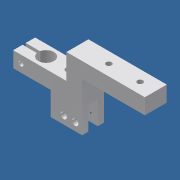
# Autodesk Inventor part: J001396
Saved by Autodesk Inventor 2012 SP2 (Build 160219200, 219)
## iProperties
Created: 2012-04-07
Part Number: J001396
Material: ALUMINUM, 6061-T651
Document SubType Name: Modeling
Designer: Igor
Density: 2.7 g/cm^3
Mass: 74.0538 g
Surface Area: 93.0623 cm^2
Volume: 27.4273 cm^3
Project: P-51601
Description: HEATER HOLDER
Vendor: HHMI: JFRC - ID&F
SPECIAL FINISH: ANODIZE PER MIL-A-8625F, TYPE II, CLASS 2 (BLACK)
ALTERED ITEM PART NUMBER: N/A
ALTERED ITEM VENDOR: N/A
DESIGN DEPARTMENT: HHMI: JFRC - ID&F
LAB/DEPT: GONEN (LAB)
REQUESTING SCIENTIST: GONEN, TAMIR
SURFACE ROUGHNESS: 32 Ra
ALTERED ITEM DESCRIPTION: N/A
Author: Igor
Revision Number: -
Autodesk Inventor part; units mm, degrees
note: some values were not read from the file. Chosen so that the rebuilt part matches the saved one: direction of "Hole3"; direction of "Hole6".
ref_plane "YZ Plane" through (0, 0, 0) normal (1, 0, 0) x (0, 1, 0)
ref_plane "XZ Plane" through (0, 0, 0) normal (0, 1, 0) x (-1, 0, 0)
ref_plane "XY Plane" through (0, 0, 0) normal (0, 0, 1) x (1, 0, 0)
sketch "Sketch1" plane through (0, 0, 0) normal (0, 0, 1) x (1, 0, 0)
  line L0 (0, 0) -> (63.5, 0)
  line L1 (63.5, 0) -> (63.5, -12.7)
  line L2 (63.5, -12.7) -> (12.7, -12.7)
  line L3 (12.7, -12.7) -> (12.7, -33.02)
  line L4 (12.7, -33.02) -> (-43.18, -33.02)
  line L5 (-43.18, -33.02) -> (-43.18, -20.32)
  line L6 (-43.18, -20.32) -> (0, -20.32)
  line L7 (0, -20.32) -> (0, 0)
  dimension "d0" = 12.7
  dimension "d2" = 12.7
  dimension "d3" = 12.7
  dimension "d4" = 43.18
  dimension "d5" = 20.32
  dimension "d22" = 50.8
  constraints: 16 end point, 6 parallel, 1 horizontal, 1 perpendicular
  measures "d0" distance of L0.end L1.end
  measures "d2" distance between parallel lines of L3 L7
  measures "d3" distance of L4.end L5.end
  measures "d4" distance between parallel lines of L7 L5
  measures "d5" distance of L6.end L0.start
  measures "d22" distance between parallel lines of L1 L3
extrude "Extrusion1" add sketch "Sketch1" along normal blind 17.78
sketch "Sketch2" plane through (0, 0, 0) normal (0, 1, 0) x (1, 0, 0)
  line L0 (63.5, 0) -> (63.5, -17.78) projected
  line L1 (0, 0) -> (0, -17.78) projected
  line L2 (0, -8.89) -> (63.5, -8.89) construction
  point P0 (50.8, -8.89)
  point P1 (25.4, -8.89)
  dimension "d8" = 12.7
  dimension "d9" = 25.4
  constraints: 2 end point, 2 midpoint, 2 point on line
  measures "d8" distance from line of L0 point (50.8, -8.89)
  measures "d9" distance of point (25.4, -8.89) point (50.8, -8.89)
hole "Hole1" at (50.8, 0, 8.89) at (25.4, 0, 8.89) direction (0, -1, 0) diameter 4.4958 end through all clearance for "Flat Head Machine Screw (82)" size "#8" standard "Ansi Unified Screw Threads"
sketch "Sketch3" plane through (-43.18, -33.02, 0) normal (0, -1, 0) x (1, 0, 0)
  line L0 (0, 0) -> (0, 17.78) projected
  line L1 (55.88, 0) -> (55.88, 17.78) projected
  line L2 (0, 8.89) -> (55.88, 8.89) construction
  arc A0 (11.5583, 7.62) -> (11.5583, 10.16) centre (17.78, 8.89) ccw
  line L3 (11.5583, 10.16) -> (0, 10.16)
  line L4 (0, 7.62) -> (11.5583, 7.62)
  line L5 (0, 10.16) -> (0, 7.62)
  point P0 (43.18, 0)
  dimension "d17" = 12.7
  dimension "d18" = 17.78
  dimension "d19" = 2.54
  constraints: 8 end point, 3 point on line, 2 midpoint, 2 point on circle, 1 centre point, 1 collinear, 1 parallel, 1 perpendicular, 1 other
  measures "d17" diameter of A0
  measures "d18" distance from line of L0 A0.centre
  measures "d19" distance between parallel lines of L4 L3
extrude "Extrusion2" cut sketch "Sketch3" against normal up to next
sketch "Sketch4" plane through (0, 0, 17.78) normal (0, 0, 1) x (1, 0, 0)
  line L0 (-43.18, -33.02) -> (-43.18, -20.32) projected
  line L1 (12.7, -12.7) -> (12.7, -33.02) projected
  line L2 (-43.18, -26.67) -> (12.7, -26.67) construction
  point P0 (-36.83, -26.67)
  dimension "d23" = 6.35
  constraints: 2 end point, 2 point on line, 1 midpoint, 1 perpendicular
  measures "d23" distance from line of point (-36.83, -26.67) L0
hole "Hole3" at (-36.83, -26.67, 17.78) direction (0, 0, -1) diameter 3.81 end up to surface clearance for "Flat Head Machine Screw (82)" size "#6" standard "Ansi Unified Screw Threads"
hole "Hole4" at (-36.83, -26.67, 17.78) direction (0, 0, -1) diameter 2.6416 end through all thread size "6-32 UNC" class "2B" standard "ANSI Unified Screw Threads"
sketch "Sketch6" plane through (-43.18, -33.02, 0) normal (0, -1, 0) x (1, 0, 0)
  line L0 (0, 10.16) -> (11.5583, 10.16) projected
  arc A0 (11.5583, 7.62) -> (11.5583, 10.16) centre (17.78, 8.89) ccw projected
  line L1 (11.5583, 7.62) -> (0, 7.62) projected
  line L2 (0, 0) -> (0, 7.62) projected
  line L3 (55.88, 0) -> (0, 0) projected
  line L4 (55.88, 0) -> (55.88, 17.78) projected
  line L5 (55.88, 17.78) -> (0, 17.78) projected
  line L6 (0, 10.16) -> (0, 17.78) projected
  line L7 (55.88, 17.78) -> (30.48, 17.78)
  line L8 (30.48, 17.78) -> (30.48, 12.7)
  line L9 (30.48, 12.7) -> (55.88, 12.7)
  line L10 (55.88, 12.7) -> (55.88, 17.78)
  line L11 (55.88, 0) -> (30.48, 0)
  line L12 (30.48, 0) -> (30.48, 5.08)
  line L13 (30.48, 5.08) -> (55.88, 5.08)
  line L14 (55.88, 5.08) -> (55.88, 0)
  point P0 (43.18, 0)
  dimension "d56" = 5.08
  dimension "d57" = 25.4
  dimension "d58" = 5.08
  dimension "d59" = 25.4
  constraints: 16 end point, 4 parallel, 2 horizontal, 2 perpendicular
  measures "d56" distance of L9.end L4.end
  measures "d57" distance between parallel lines of L8 L4
  measures "d58" distance between parallel lines of L3 L13
  measures "d59" distance between parallel lines of L12 L14
extrude "Extrusion3" add sketch "Sketch6" along normal blind 19.05 contours L5 L4 L9 L8 | L12 L13 L4 L3
sketch "Sketch8" plane through (0, 0, 17.78) normal (0, 0, 1) x (1, 0, 0)
  line L0 (-12.7, -33.02) -> (-43.18, -33.02) projected
  line L1 (12.7, -12.7) -> (12.7, -52.07) projected
  point P0 (0, 0)
  point P1 (7.112, -45.72)
  point P2 (-2.286, -45.72)
  dimension "d66" = 12.7
  dimension "d67" = 12.7
  dimension "d68" = 14.986
  dimension "d69" = 9.398
  measures "d66" distance from line of L0 point (-2.286, -45.72)
  measures "d67" distance from line of L0 point (7.112, -45.72)
  measures "d68" distance from line of point (-2.286, -45.72) L1
  measures "d69" distance of point (7.112, -45.72) point (-2.286, -45.72)
hole "Hole6" at (7.112, -45.72, 17.78) at (-2.286, -45.72, 17.78) direction (0, 0, -1) diameter 5.08 end up to surface
hole "Hole7" at (-2.286, -45.72, 17.78) direction (0, 0, -1) diameter 1.7018 end through all
hole "Hole8" at (7.112, -45.72, 17.78) direction (0, 0, -1) diameter 1.7018 end through all
sketch "Sketch9" plane through (-43.18, -20.32, 0) normal (0, 1, 0) x (1, 0, 0)
  line L0 (11.5583, -10.16) -> (0, -10.16) projected
  line L1 (0, -10.16) -> (0, -17.78) projected
  line L2 (0, -17.78) -> (43.18, -17.78) projected
  line L3 (43.18, 0) -> (43.18, -17.78) projected
  line L4 (0, 0) -> (43.18, 0) projected
  line L5 (0, 0) -> (0, -7.62) projected
  line L6 (0, -7.62) -> (11.5583, -7.62) projected
  arc A0 (11.5583, -10.16) -> (11.5583, -7.62) centre (17.78, -8.89) ccw projected
  point P0 (36.195, -8.89)
  dimension "d95" = 18.415
  measures "d95" distance of point (36.195, -8.89) A0.centre
hole "Hole9" at (-6.985, -20.32, 8.89) direction (0, -1, 0) diameter 5.08 end through all
equation "\"d67\" = d66"
body "Solid1"
